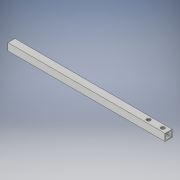
# Autodesk Inventor part: arm
Saved by Autodesk Inventor 2019 (Build 230136000, 136)
## iProperties
Created: 2019-02-02
Part Number: arm
Material: Generic
Document SubType Name: Modeling
Designer: suchanek
Density: 1 g/cm^3
Appearance: Default
Author: suchanek
Autodesk Inventor part; units mm, degrees
ref_plane "YZ Plane" through (0, 0, 0) normal (1, 0, 0) x (0, 1, 0)
ref_plane "XZ Plane" through (0, 0, 0) normal (0, 1, 0) x (-1, 0, 0)
ref_plane "XY Plane" through (0, 0, 0) normal (0, 0, 1) x (1, 0, 0)
sketch "Sketch1" plane through (0, 0, 0) normal (1, 0, 0) x (0, 1, 0)
  line L0 (-5, 5) -> (5, 5)
  line L1 (5, 5) -> (5, -5)
  line L2 (5, -5) -> (-5, -5)
  line L3 (-5, -5) -> (-5, 5)
  line L4 (-5, 5) -> (5, -5) construction
  line L5 (5, 5) -> (-5, -5) construction
  line L6 (-4, 4) -> (4, 4)
  line L7 (4, 4) -> (4, -4)
  line L8 (4, -4) -> (-4, -4)
  line L9 (-4, -4) -> (-4, 4)
  line L10 (-4, 4) -> (4, -4) construction
  line L11 (4, 4) -> (-4, -4) construction
  point P0 (0, 0)
  dimension "d0" = 10
  dimension "d1" = 10
  dimension "d2" = 8
  dimension "d3" = 8
  constraints: 24 end point, 4 midpoint, 4 parallel, 2 horizontal, 2 perpendicular
  measures "d0" distance of L1.end L2.end
  measures "d1" distance of L0.end L1.end
  measures "d2" distance of L7.end L8.end
  measures "d3" distance of L6.end L7.end
extrude "Extrusion1" add sketch "Sketch1" along normal blind 220
sketch "Sketch2" plane through (0, 5, 5) normal (0, 1, 0) x (1, 0, 0)
  circle A0 centre (212, 5) radius 2.6
  line L0 (220, 10) -> (220, 0) projected
  circle A1 centre (192, 5) radius 2.6
  line L1 (0, 0) -> (220, 0) projected
  point P0 (0, 5)
  dimension "d8" = 5.2
  dimension "d9" = 8
  dimension "d10" = 5.2
  dimension "d11" = 20
  dimension "d12" = 5
  constraints: 2 centre point, 1 horizontal alignment
  measures "d8" diameter of A0
  measures "d9" distance from line of L0 A0.centre
  measures "d10" diameter of A1
  measures "d11" distance of A0.centre A1.centre
  measures "d12" distance from line of L1 A0.centre
extrude "Extrusion2" cut sketch "Sketch2" against normal blind 10
body "Solid1"
